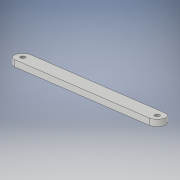
# Autodesk Inventor part: 連接6
Saved by Autodesk Inventor 2017 (Build 210142000, 142)
## iProperties
Part Number: 連接6
Material: 一般
Document SubType Name: Modeling
Designer: User
Density: 1 g/cm^3
Appearance: 預設
Author: User
Autodesk Inventor part; units mm, degrees
ref_plane "YZ Plane" through (0, 0, 0) normal (1, 0, 0) x (0, 1, 0)
ref_plane "XZ Plane" through (0, 0, 0) normal (0, 1, 0) x (-1, 0, 0)
ref_plane "XY Plane" through (0, 0, 0) normal (0, 0, 1) x (1, 0, 0)
sketch "草圖1" plane through (0, 0, 0) normal (0, 1, 0) x (-1, 0, 0)
  circle A0 centre (0, 0) radius 1.25
  line L0 (0, 0) -> (-80, 0)
  circle A1 centre (-80, 0) radius 1.25
  circle A2 centre (-80, 0) radius 4
  circle A3 centre (0, 0) radius 4
  line L1 (0, 4) -> (-80, 4)
  line L2 (-80, -4) -> (0, -4)
  dimension "d0" = 2.5
  dimension "d14" = 80
  dimension "d15" = 2.5
  dimension "d16" = 8
  dimension "d17" = 8
  constraints: 6 end point, 4 centre point, 4 coincident, 4 point on circle, 3 tangent, 2 horizontal
  measures "d0" diameter of A0
  measures "d14" distance of L0.start L0.end
  measures "d15" diameter of A1
  measures "d16" diameter of A2
  measures "d17" diameter of A3
extrude "擠出1" add sketch "草圖1" along normal mid plane 3
sketch "草圖2" plane through (0, 1.5, 0) normal (0, 1, 0) x (1, 0, 0)
  circle A0 centre (80, 0) radius 1.5 projected
  circle A1 centre (0, 0) radius 1.25 projected
  arc A2 (0, 6) -> (0, -6) centre (0, 0) ccw projected
  line L0 (0, -6) -> (80, -6) projected
  arc A3 (80, -6) -> (80, 6) centre (80, 0) ccw projected
  line L1 (80, 6) -> (0, 6) projected
  line L2 (80, 0) -> (70, 0)
  line L3 (70, 0) -> (70, 1.5)
  line L4 (70, 1.5) -> (62.5, 1.5)
  line L5 (62.5, 1.5) -> (62.5, -1.5)
  line L6 (62.5, -1.5) -> (70, -1.5)
  line L7 (70, -1.5) -> (70, 0)
  line L8 (62.5, 0) -> (48, 0)
  circle A4 centre (48, 0) radius 1.5
  line L9 (48, 0) -> (15, 0)
  line L10 (15, 0) -> (15, 1.5)
  line L11 (15, 1.5) -> (10, 1.5)
  line L12 (10, 1.5) -> (10, -1.5)
  line L13 (10, -1.5) -> (15, -1.5)
  line L14 (15, -1.5) -> (15, 0)
  dimension "d18" = 10
  dimension "d19" = 1.5
  dimension "d20" = 7.5
  dimension "d21" = 3
  dimension "d22" = 14.5
  dimension "d23" = 3
  dimension "d24" = 33
  dimension "d25" = 1.5
  dimension "d26" = 5
  dimension "d27" = 3
  constraints: 26 end point, 9 perpendicular, 3 horizontal, 2 point on line, 1 centre point, 1 coincident, 1 midpoint, 1 parallel
  measures "d18" distance of L2.start L2.end
  measures "d19" distance of L2.end L3.end
  measures "d20" distance of L3.end L4.end
  measures "d21" distance of L4.end L5.end
  measures "d22" distance of L8.start L8.end
  measures "d23" diameter of A4
  measures "d24" distance of L9.start L9.end
  measures "d25" distance of L9.end L10.end
  measures "d26" distance of L10.end L11.end
  measures "d27" distance of L11.end L12.end
